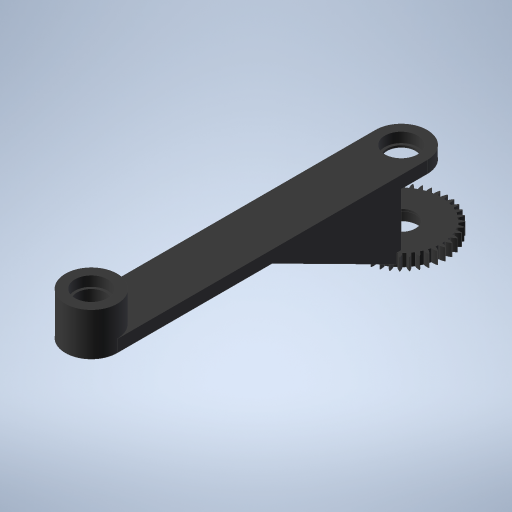
# Autodesk Inventor part: inner arm
Saved by Autodesk Inventor 2024 (Build 280153000, 153)
## iProperties
Created: 2024-04-04
Part Number: inner arm
Material: Generic
Document SubType Name: Modeling
Designer: drew
Density: 1 g/cm^3
Appearance: Default
Author: drew
Autodesk Inventor part; units mm, degrees
ref_plane "YZ Plane" through (0, 0, 0) normal (1, 0, 0) x (0, 1, 0)
ref_plane "XZ Plane" through (0, 0, 0) normal (0, 1, 0) x (-1, 0, 0)
ref_plane "XY Plane" through (0, 0, 0) normal (0, 0, 1) x (1, 0, 0)
sketch "Sketch1" plane through (0, 0, 0) normal (0, 1, 0) x (-1, 0, 0)
  line L0 (0, 76.2) -> (0, -76.2) construction
  line L1 (-12.7, 76.2) -> (-12.7, -76.2)
  line L2 (12.7, -76.2) -> (12.7, 76.2)
  arc A0 (12.7, 76.2) -> (-12.7, 76.2) centre (0, 76.2) ccw
  arc A1 (-12.7, -76.2) -> (12.7, -76.2) centre (0, -76.2) ccw
  circle A2 centre (0, -76.2) radius 7
  circle A3 centre (0, 76.2) radius 7
  point P0 (0, 0)
  dimension "d0" = 76.2
  dimension "d1" = 25.4
  dimension "d2" = 14
  dimension "d3" = 14
  constraints: 8 end point, 4 centre point, 4 point on circle, 4 tangent, 2 coincident, 1 midpoint, 1 parallel, 1 vertical
  measures "d0" distance of point (0, 0) L0.end
  measures "d1" diameter of A1
  measures "d2" diameter of A2
  measures "d3" diameter of A3
extrude "Extrusion1" add sketch "Sketch1" along normal blind 38.1
sketch "Sketch2" plane through (12.7, 0, 76.2) normal (1, 0, 0) x (0, 0, -1)
  line L0 (0, 0) -> (152.4, 0) projected
  line L1 (152.4, 0) -> (152.4, 38.1) projected
  line L2 (0, 38.1) -> (152.4, 38.1) projected
  line L3 (0, 0) -> (0, 38.1) projected
  line L4 (0, 0) -> (0, 0) projected
  line L5 (0, 0) -> (0, 38.1) projected
  line L6 (0, 38.1) -> (0, 38.1) projected
  line L7 (0, 0) -> (0, 38.1) projected
  line L8 (165.1, 0) -> (165.1, 38.1) projected
  line L9 (-12.7, 0) -> (-12.7, 38.1) projected
  line L10 (139.7, 38.1) -> (139.7, 0) construction
  line L11 (76.2, 38.1) -> (76.2, 0) construction
  line L12 (139.7, 0) -> (76.2, 32.1)
  line L13 (76.2, 32.1) -> (-12.7, 32.1)
  line L14 (-12.7, 0) -> (0, 0)
  dimension "d6" = 25.4
  dimension "d7" = 6
  constraints: 10 end point, 4 point on line, 2 perpendicular, 1 horizontal, 1 midpoint, 1 vertical
  measures "d6" distance between parallel lines of L8 L10
  measures "d7" distance from line of L2 L12.end
extrude "Extrusion2" cut sketch "Sketch2" against normal through all contours L3 L13 L12 L0 | L14 L9 L13 L3
sketch "Sketch3" plane through (0, 38.1, 0) normal (0, 1, 0) x (1, 0, 0)
  circle A0 centre (0, -76.2) radius 7 projected
  circle A1 centre (0, 76.2) radius 7 projected
  circle A2 centre (0, -76.2) radius 8.1
  circle A3 centre (0, 76.2) radius 8.1
  point P0 (0, 0)
  dimension "d10" = 16.2
  dimension "d11" = 16.2
  constraints: 2 centre point, 2 coincident
  measures "d10" diameter of A2
  measures "d11" diameter of A3
extrude "Extrusion3" cut sketch "Sketch3" against normal blind 5 contours A1 | A3
sketch "Sketch4" plane through (0, 0, 0) normal (0, -1, 0) x (1, 0, 0)
  circle A0 centre (0, -76.2) radius 8.1 projected
  point P0 (0, 0)
extrude "Extrusion4" cut sketch "Sketch4" against normal blind 5
sketch "Sketch5" plane through (12.7, 0, -76.2) normal (1, 0, 0) x (0, 0, -1)
  line L0 (-12.7, 6) -> (-12.7, 32.1)
  line L1 (-12.7, 32.1) -> (12.7, 32.1)
  line L2 (12.7, 32.1) -> (12.7, 6)
  line L3 (12.7, 6) -> (-12.7, 6)
  line L4 (-152.4, 38.1) -> (0, 38.1) projected
  line L5 (-12.7, 0) -> (0, 0) projected
  point P0 (-76.2, 0)
  dimension "d16" = 6
  dimension "d17" = 6
  dimension "d18" = 25.4
  constraints: 8 end point, 2 perpendicular, 1 parallel, 1 point on line, 1 vertical
  measures "d16" distance between parallel lines of L4 L1
  measures "d17" distance between parallel lines of L5 L3
  measures "d18" distance between parallel lines of L2 L0
extrude "Extrusion5" cut sketch "Sketch5" against normal blind 25.4
sketch "Sketch6" plane through (0, 0, 0) normal (1, 0, 0) x (0, 1, 0)
  line L0 (6, -63.5) -> (32.1, -63.5) projected
  line L1 (6, -76.2) -> (6, -88.9) projected
  line L2 (32.1, -59.69) -> (6, -59.69)
  line L3 (6, -59.69) -> (6, -76.2)
  line L4 (6, -76.2) -> (32.1, -76.2)
  line L5 (32.1, -76.2) -> (32.1, -59.69)
  line L6 (45.72, -76.2) -> (-7.62, -76.2) projected
  point P0 (0, 0)
  dimension "d21" = 16.51
  constraints: 8 end point, 2 parallel, 1 horizontal, 1 perpendicular
  measures "d21" distance between parallel lines of L4 L2
revolve "Revolution1" cut sketch "Sketch6" angle 360 about axis through (0, 38.1, -76.2) along (0, -1, 0)
sketch "Sketch7" plane through (0, 0, 0) normal (0, -1, 0) x (1, 0, 0)
  circle A0 centre (0, -76.2) radius 8.1 projected
  circle A1 centre (0, -76.2) radius 21.1667 construction
  line L0 (0, -76.2) -> (21.1667, -76.2) construction
  line L1 (21.1667, -76.2) -> (21.1667, -56.5953) construction
  line L2 (21.1667, -76.2) -> (24.3155, -84.8514) construction
  line L3 (0, -76.2) -> (18.6906, -69.3972) construction
  circle A2 centre (0, -76.2) radius 19.8902 construction
  arc A3 (18.6906, -69.3972) -> (16.411, -64.9618) centre (0, -76.2) ccw
  line L4 (16.411, -64.9618) -> (0, -76.2) construction
  line L5 (14.7298, -62.5067) -> (23.3265, -75.0604) construction
  arc A4 (19.6728, -73.2678) -> (18.6906, -69.3972) centre (0, -76.2) ccw
  line L6 (19.6728, -73.2678) -> (19.6728, -73.2678) construction
  line L7 (19.6728, -73.2678) -> (20.1504, -76.4718) construction
  arc A5 (19.888, -76.4964) -> (18.6906, -69.3972) centre (0, -76.2) ccw
  point P0 (0, 0)
  dimension "d23" = 42.3333
  dimension "d24" = 20
  dimension "d25" = 7.2394
  dimension "d28" = 5
  dimension "d29" = 12.2394
  dimension "d30" = 4
  dimension "d32" = 3.2394
  dimension "d33" = 7.2394
  constraints: 16 end point, 8 point on circle, 6 tangent, 5 point on line, 4 centre point, 4 coincident, 1 concentric, 1 horizontal, 1 horizontal alignment, 1 perpendicular, 1 vertical, 2 other
  measures "d24" angle of L1 L2
  measures "d25" distance of L0.end L3.end
  measures "d29" distance of L5.end L4.start
  measures "d32" distance of L6.end L7.end
sketch "Sketch8" plane through (0, 0, 0) normal (0, -1, 0) x (1, 0, 0)
  spline S0 degree 3 poles (23.3265, -75.0604) (21.8696, -76.156) (20.2087, -76.5115) (19.888, -76.4964) knots 0 0 0 0 1 1 1 1
  line L0 (0, -76.2) -> (21.4301, -75.6777) construction
  line L1 (19.888, -76.4964) -> (0, -76.2) construction
  spline S1 degree 3 poles (23.3543, -76.202) (21.8458, -75.1787) (20.1696, -74.9045) (19.8499, -74.9351) knots 0 0 0 0 1 1 1 1
  circle A0 centre (0, -76.2) radius 22.225
  line L2 (19.888, -76.4964) -> (19.638, -76.4927)
  arc A1 (19.638, -76.4927) -> (19.6343, -75.7215) centre (0, -76.2) ccw
  line L3 (19.8499, -74.9351) -> (19.6004, -74.951)
  arc A2 (19.6343, -75.7215) -> (19.6004, -74.951) centre (0, -76.2) ccw
  circle A3 centre (0, -76.2) radius 19.6402
  point P0 (0, 0)
  point P1 (21.1667, -76.2)
  point P2 (20.1504, -76.4718)
  point P3 (21.1415, -75.1689)
  point P4 (20.1132, -74.947)
  dimension "d34" = 2.25
  dimension "d35" = 44.45
  dimension "d36" = 0.25
  constraints: 8 end point, 5 symmetric about line, 4 centre point, 4 coincident, 4 point on circle, 2 point on line, 1 concentric, 9 other
  measures "d34" angle of L1 L0
  measures "d35" diameter of A0
  measures "d36" distance of L2.end L1.start
sketch "Sketch9" plane through (0, 0, 0) normal (0, -1, 0) x (1, 0, 0)
  circle A0 centre (0, -76.2) radius 19.6402 projected
  circle A1 centre (0, -76.2) radius 8.1 projected
  point P0 (0, 0)
extrude "Extrusion6" add sketch "Sketch9" against normal up to surface (6 mm away)
sketch "Sketch10" plane through (0, 0, -76.2) normal (0, -1, 0) x (1, 0, 0)
  spline S0 degree 3 poles (23.3543, -0.002) (21.8458, 1.0213) (20.1696, 1.2955) (19.8499, 1.2649) knots 0 0 0 0 1 1 1 1 projected
  line L0 (19.8499, 1.2649) -> (19.6004, 1.249) projected
  arc A0 (19.6343, 0.4785) -> (19.6004, 1.249) centre (0, 0) ccw projected
  arc A1 (19.638, -0.2927) -> (19.6343, 0.4785) centre (0, 0) ccw projected
  spline S1 degree 3 poles (23.3265, 1.1396) (21.8696, 0.044) (20.2087, -0.3115) (19.888, -0.2964) knots 0 0 0 0 1 1 1 1 projected
  circle A2 centre (0, 0) radius 22.225 projected
  line L1 (19.888, -0.2964) -> (0, 0) construction
  line L2 (19.638, -0.2927) -> (19.888, -0.2964)
  point P0 (0, 76.2)
  point P1 (22.2204, 0.4513)
  point P2 (22.216, 0.6317)
  constraints: 2 end point
extrude "Extrusion7" add sketch "Sketch10" against normal up to surface (6 mm away) contours A2 S1 L2 A1 A0 L0 S0 picked at (21.3131, 0.5294)
pattern_circular "Circular Pattern1" count 40 over 360 about axis through (0, 38.1, -76.2) along (0, -1, 0) of "Extrusion7"
sketch "Sketch11" plane through (0, 38.1, 0) normal (0, 1, 0) x (1, 0, 0)
  circle A0 centre (0, -76.2) radius 7 projected
  arc A1 (-12.7, -76.2) -> (12.7, -76.2) centre (0, -76.2) ccw projected
  circle A2 centre (0, -76.2) radius 12.7
  point P0 (0, 0)
  point P1 (12.7, -76.2)
  constraints: 1 coincident, 3 other
extrude "Extrusion8" add sketch "Sketch11" along normal blind 15
sketch "Sketch12" plane through (0, 53.1, 76.2) normal (0, 1, 0) x (1, 0, 0)
  circle A0 centre (0, 0) radius 7 projected
  circle A1 centre (0, 0) radius 8.1
  point P0 (0, 76.2)
  dimension "d46" = 16.2
  constraints: 1 centre point, 1 coincident
  measures "d46" diameter of A1
extrude "Extrusion9" cut sketch "Sketch12" against normal blind 5
sketch "Sketch13" plane through (12.7, 32.1, 0) normal (0, -1, 0) x (1, 0, 0)
  circle A0 centre (-12.7, 76.2) radius 8.1 projected
  circle A1 centre (-12.7, 76.2) radius 7 projected
  point P0 (-12.7, 0)
extrude "Extrusion10" cut sketch "Sketch13" against normal blind 5
equation "\"d29\" = d25 + d28"
equation "\"d32\" = d25 - d30"
equation "\"d33\" = d25"
equation "\"d35\" = dia + 2 * mod"
equation "\"mod\" = 1.05833"
equation "\"dia\" = 42.33333"
body "Solid1"
